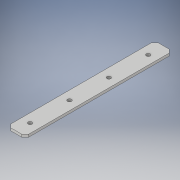
# Autodesk Inventor part: vin
Saved by Autodesk Inventor 2019 (Build 230136000, 136)
## iProperties
Created: 2019-07-08
Part Number: vin
Material: Ogólny
Document SubType Name: Modeling
Designer: Kurat
Density: 1 g/cm^3
Appearance: Domyślna
Author: Kurat
Autodesk Inventor part; units mm, degrees
ref_plane "YZ Plane" through (0, 0, 0) normal (1, 0, 0) x (0, 1, 0)
ref_plane "XZ Plane" through (0, 0, 0) normal (0, 1, 0) x (-1, 0, 0)
ref_plane "XY Plane" through (0, 0, 0) normal (0, 0, 1) x (1, 0, 0)
sketch "Szkic1" plane through (0, 0, 0) normal (0, 1, 0) x (-1, 0, 0)
  line L0 (8.89, -1.91) -> (8.89, -57.14)
  line L1 (6.98, -59.05) -> (1.91, -59.05)
  line L2 (0, -57.14) -> (0, -1.91)
  line L3 (6.98, 0) -> (8.89, -1.91)
  line L4 (1.91, 0) -> (0, -1.91)
  line L5 (0, -57.14) -> (1.91, -59.05)
  line L6 (6.98, -59.05) -> (8.89, -57.14)
  line L7 (6.98, 0) -> (1.91, 0)
  line L8 (4.445, -59.05) -> (4.445, 0)
  circle A0 centre (4.445, -6.35) radius 0.75
  circle A1 centre (4.445, -21.59) radius 0.75
  circle A2 centre (4.445, -36.83) radius 0.75
  circle A3 centre (4.445, -52.07) radius 0.75
  line L9 (7.89, -56.7258) -> (6.5658, -58.05)
  line L10 (6.5658, -58.05) -> (2.3242, -58.05)
  line L11 (2.3242, -58.05) -> (1, -56.7258)
  line L12 (1, -56.7258) -> (1, -2.3242)
  line L13 (1, -2.3242) -> (2.3242, -1)
  line L14 (2.3242, -1) -> (6.5658, -1)
  line L15 (6.5658, -1) -> (7.89, -2.3242)
  line L16 (7.89, -2.3242) -> (7.89, -56.7258)
  point P0 (0, 0)
  point P1 (8.89, -59.05)
  point P2 (8.89, 0)
  point P3 (0, -59.05)
  dimension "d0" = 8.89
  dimension "d2" = 1.91
  dimension "d3" = 1.91
  dimension "d4" = 1.91
  dimension "d5" = 1.91
  dimension "d6" = 1.91
  dimension "d7" = 1.91
  dimension "d8" = 1.91
  dimension "d9" = 1.91
  dimension "d10" = 1.5
  dimension "d11" = 6.35
  dimension "d14" = 15.24
  dimension "d19" = 1
  constraints: 34 end point, 7 point on line, 4 centre point, 2 midpoint, 2 parallel, 1 vertical, 13 other
  measures "d0" distance of point (8.89, -59.05) point (0, -59.05)
  measures "d2" distance of L3.start point (8.89, 0)
  measures "d3" distance of L0.start point (8.89, 0)
  measures "d4" distance of L4.start point (0, 0)
  measures "d5" distance of L2.end point (0, 0)
  measures "d6" distance of L2.start point (0, -59.05)
  measures "d7" distance of L1.end point (0, -59.05)
  measures "d8" distance of L1.start point (8.89, -59.05)
  measures "d9" distance of L0.end point (8.89, -59.05)
  measures "d10" diameter of A0
  measures "d11" distance of L8.end A0.centre
  measures "d14" distance of A0.centre A1.centre
  measures "d19" distance between parallel lines of L0 L16
extrude "Wyciągnięcie proste1" add sketch "Szkic1" along normal blind 1 contours L14 L15 L16 L9 L10 L8 A3 A2 A1 A0 | L8 A0 A1 A2 A3 L10 L11 L12 L13 L14
equation "\"d3\" = d2"
equation "\"d4\" = d2"
equation "\"d5\" = d4"
equation "\"d6\" = d2"
equation "\"d7\" = d6"
equation "\"d8\" = d2"
equation "\"d9\" = d8"
